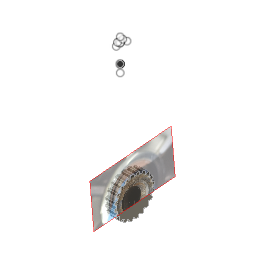
test spline 30 v1 (Autodesk Fusion 360 design; units mm, degrees)
Autodesk Fusion 360 part; units mm, degrees
note: some values were not read from the file. Chosen so that the rebuilt part matches the saved one: which face or edge a step refers to.
sketch "Sketch1" plane through (0, 0, 0) normal (1, 0, 0) x (0, 1, 0)
  circle A0 centre (0, 0) radius 10.552 construction
  line L0 (0, 0) -> (0, -4.2525) construction
  line L1 (-1.3499, 11.279) -> (0, 9.3148)
  line L2 (0, 9.3148) -> (1.3499, 11.279)
  arc A1 (3.7731, 8.9842) -> (-2.171, 9.4995) centre (0, 0) ccw
  arc A2 (0.4007, 9.8979) -> (-0.4007, 9.8979) centre (0, 0) ccw
  line L3 (0, 0) -> (0.8279, 10.5194) construction
  line L4 (0, 0) -> (-0.8279, 10.5194) construction
  line L5 (0.8279, 10.5194) -> (0.3632, 10.8388) construction
  line L6 (-0.8279, 10.5194) -> (-0.4118, 10.8054) construction
  line L7 (0.8279, 10.5194) -> (0.3009, 10.5609) construction
  line L8 (-0.8279, 10.5194) -> (-0.4014, 10.553) construction
  circle A3 centre (0, 0) radius 11.0365
  circle A4 centre (-0.1808, 9.9581) radius 0.2153
  circle A5 centre (0.1808, 9.9581) radius 0.2153
  circle A6 centre (0, 0) radius 11.3595
  circle A7 centre (-1.4532, 11.049) radius 0.2153
  circle A8 centre (1.4532, 11.049) radius 0.2153
  line L9 (0, 9.3148) -> (0, 12.8891) construction
  dimension "d1" = 21.1039
  dimension "d8" = 9.7444
  dimension "d9" = 9.906
  dimension "d26" = 9
  dimension "d28" = 30
  dimension "d29" = 37.5
  dimension "d32" = 22.073
  dimension "d41" = 0.4307
  dimension "d42" = 22.719
  dimension "d43" = 69
  constraint coincident A0.centre L0.start
  constraint vertical L0
  constraint coincident A0 L4.end
  constraint coincident A0 L3.end
  constraint symmetric L0 L3.end L4.end
  constraint coincident L2 L3.end
  constraint coincident L1 L4.end
  constraint coincident L1.end L2.start
  constraint coincident L0 L1.end
  constraint perpendicular L2 L5
  constraint perpendicular L1 L6
  constraint tangent A0 L8
  constraint tangent A0 L7
  constraint equal A4 A5
  constraint coincident L2.end A6
  constraint coincident L1.start A6
  constraint equal A4 A8
  constraint equal A4 A7
  constraint vertical L9
  constraint coincident L1 A2.end
  constraint coincident L2 A2.start
  constraint tangent A1 A4
  constraint tangent A1 A5
  constraint tangent L2 A5
  constraint tangent L1 A4
  constraint tangent A6 A7
  constraint tangent L1 A7
  constraint tangent L2 A8
  constraint tangent A6 A8
  measures "d1" diameter of A0
  measures "d8" radius of A1
  measures "d9" radius of A2
  measures "d26" angle of L3 L4
  measures "d28" angle of L5 L7
  measures "d32" diameter of A3
  measures "d41" diameter of A4
  measures "d42" diameter of A6
  measures "d43" angle of L1 L2
sketch "Sketch2" plane through (0, 0, 0) normal (1, 0, 0) x (0, 1, 0)
  circle A0 centre (0, 0) radius 11.0365
  arc A1 (3.7731, 8.9842) -> (-2.171, 9.4995) centre (0, 0) ccw
  line L0 (0, 9.3148) -> (1.3499, 11.279)
  line L1 (-1.3499, 11.279) -> (0, 9.3148)
  dimension "d31" = 22.073
  constraint coincident A0.centre A1.centre
  measures "d31" diameter of A0
extrude "Extrude1" add sketch "Sketch1" sketch "Sketch2" along normal blind 5 contours L1 A1 A4 | L1 L2 A1 | L2 A1 A5 of sketch 2 contours A0 L0 L1
pattern_circular "C-Pattern1" count 20 over 360 about axis through (1.75, 0, 0) along (1, 0, 0) of 5 faces at (1.6667, 0.6197, 10.2165) (3.3333, -0.0197, 9.7444) (1.6667, -0.3524, 9.8279) (3.3333, 0.3524, 9.8279) (1.6667, -0.8811, 10.5968)
move_body "Move1" bodies 1 to x (1, 0, 0) y (0, 1, 0) z (0, 0, 1) at (0, 1.8731, -53.0546)
move_body "Move2" bodies 1 to x (1, 0, 0) y (0, 1, 0) z (0, 0, 1) at (0, 1, -9)
move_body "Move3" bodies 1 to x (1, 0, 0) y (0, 0.999391, -0.034899) z (0, 0.034899, 0.999391) at (0, 2.1674, 0.0625)
equation "modulus = 1.0767 mm" comment "modulus"
equation "D2 = 21.1039 mm" comment "Diameter modulus"
equation "d41 = modulus * 0.4"
